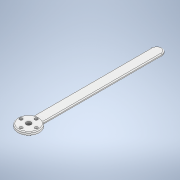
# Autodesk Inventor part: base2
Saved by Autodesk Inventor 2022 (Build 260153000, 153)
## iProperties
Created: 2022-06-14
Part Number: base2
Material: ABS プラスチック
Document SubType Name: Modeling
Designer: yuto6
Density: 1.06 g/cm^3
Appearance: 滑らか - 白
Author: yuto6
Autodesk Inventor part; units mm, degrees
ref_plane "YZ Plane" through (0, 0, 0) normal (1, 0, 0) x (0, 1, 0)
ref_plane "XZ Plane" through (0, 0, 0) normal (0, 1, 0) x (-1, 0, 0)
ref_plane "XY Plane" through (0, 0, 0) normal (0, 0, 1) x (1, 0, 0)
sketch "スケッチ1" plane through (0, 0, 0) normal (0, 1, 0) x (-1, 0, 0)
  circle A0 centre (0, 0) radius 12
  line L0 (0, 0) -> (6, 0)
  line L1 (6, 0) -> (6, -150)
  line L2 (6, -150) -> (0, -150)
  line L3 (0, -150) -> (0, 0)
  point P0 (6, -10.3923)
  point P1 (0, -12)
  dimension "d0" = 24
  dimension "d3" = 150
  dimension "d4" = 6
  constraints: 8 end point, 2 parallel, 1 centre point, 1 coincident, 1 horizontal, 1 perpendicular
  measures "d0" diameter of A0
  measures "d3" distance of L0.end L1.end
  measures "d4" distance of L1.end L2.end
extrude "押し出し1" add sketch "スケッチ1" along normal blind 4 contours A0 L1 L0 L3 | L3 L0 L1 A0
sketch "スケッチ2" plane through (0, 4, 0) normal (0, 1, 0) x (1, 0, 0)
  circle A0 centre (0, 0) radius 8.5
  point P0 (-8.5, 0)
  dimension "d5" = 17
  constraints: 1 coincident, 1 horizontal alignment, 2 other
hole "穴1" at (-8.5, 4, 0) direction (0, -1, 0) diameter 3.4 end through all clearance for "Flat Head Machine Screw" size "M3" standard "Ansi Metric M Profile"
pattern_circular "円形状パターン1" count 4 over 360 about axis through (0, 0, 0) along (0, 1, 0) of "穴1"
extrude "押し出し2" add sketch "スケッチ1" along normal blind 3 contours A0 L1 L2 L3
mirror "ミラー1" about plane through (0, 0, 0) normal (1, 0, 0) of "押し出し2"
sketch "スケッチ3" plane through (0, 4, 0) normal (0, 1, 0) x (1, 0, 0)
  point P0 (0, 0)
hole "穴2" at (0, 4, 0) direction (0, -1, 0) diameter 5.5 end through all clearance for "Flat Head Machine Screw" size "M5" standard "Ansi Metric M Profile"
fillet "フィレット2" radius 6 2 edges at (-6, 1.5, -150) (6, 1.5, -150)
fillet "フィレット1" radius 1 9 edges at (-6, 3, -77.1962) (6, 3, -77.1962) (12, 4, 0) (6, 0, 10.3923) (-10.3923, 0, -6) (-6, 0, -77.1962) (6, 0, -77.1962) (0, 3, -150) (0, 0, -150)
